Autodesk Fusion 360 part; units mm, degrees
note: some values were not read from the file. Chosen so that the rebuilt part matches the saved one: which bodies a step acts on.
(part 2 of 2)
sketch "Esquisse264" plane through (0, 25.75, 0) normal (0, 1, 0) x (1, 0, 0)
  spline S0 degree 5 poles (123.1631, -52) (123.1652, -52.1666) (123.167, -52.4997) (123.1624, -52.9994) (123.1419, -53.6656) (123.0924, -54.4971) (123.0197, -55.3268) (122.9244, -56.1541) (122.8078, -56.9784) (122.6713, -57.7994) (122.5162, -58.6168) (122.3444, -59.4305) (122.1576, -60.2403) (121.9575, -61.0465) (121.7457, -61.8491) (121.5239, -62.6484) (121.2935, -63.4447) (121.0557, -64.2383) (120.8113, -65.0295) (120.561, -65.8186) (120.305, -66.6056) (120.0432, -67.3906) (119.7752, -68.1736) (119.5004, -68.9543) (119.2175, -69.7325) (118.9255, -70.5075) (118.6227, -71.2788) (118.3076, -72.0454) (117.9784, -72.8065) (117.6337, -73.5608) (117.2717, -74.3073) (116.891, -75.0446) (116.4903, -75.7713) (116.0688, -76.4862) (115.6257, -77.188) (115.1609, -77.8756) (114.6743, -78.548) (114.1664, -79.2042) (113.638, -79.8439) (113.0901, -80.4668) (112.5241, -81.073) (111.9416, -81.6629) (111.3444, -82.2371) (110.7343, -82.7967) (110.1134, -83.3429) (109.4834, -83.8772) (108.8464, -84.4013) (108.2041, -84.9169) (107.558, -85.4257) (106.9097, -85.9295) (106.2604, -86.4299) (105.6109, -86.9284) (104.9621, -87.4261) (104.3142, -87.9239) (103.6674, -88.4223) (103.0212, -88.9214) (102.3753, -89.4209) (101.7287, -89.9203) (101.0804, -90.4184) (100.4293, -90.914) (99.7739, -91.4054) (99.113, -91.8906) (98.4451, -92.3676) (97.7689, -92.834) (97.0833, -93.2877) (96.3873, -93.7262) (95.6801, -94.1472) (94.9613, -94.5486) (94.2307, -94.9285) (93.4883, -95.2851) (92.7345, -95.617) (91.9699, -95.9233) (91.1952, -96.2031) (90.4115, -96.4564) (89.6197, -96.6831) (88.821, -96.8839) (88.0167, -97.0597) (87.2077, -97.2118) (86.3953, -97.3415) (85.5803, -97.4507) (84.7636, -97.541) (83.946, -97.6145) (83.128, -97.6729) (82.31, -97.7181) (81.4926, -97.7516) (80.6758, -97.7751) (79.8598, -97.7897) (79.0447, -97.7964) (78.2305, -97.7959) (77.4172, -97.7887) (76.6046, -97.7748) (75.7929, -97.7541) (74.9819, -97.7263) (74.1716, -97.6907) (73.3619, -97.6467) (72.5531, -97.5936) (71.7452, -97.5305) (70.9382, -97.4567) (70.1325, -97.3715) (69.3281, -97.2746) (68.5253, -97.1656) (67.7242, -97.0445) (66.925, -96.9115) (66.1277, -96.7671) (65.3324, -96.6119) (64.539, -96.4469) (63.7472, -96.2733) (62.9567, -96.0923) (62.1673, -95.9052) (61.3784, -95.7135) (60.5895, -95.5184) (59.8001, -95.3212) (59.0096, -95.1228) (58.2176, -94.9242) (57.4236, -94.7256) (56.6273, -94.5271) (55.8285, -94.3286) (55.0272, -94.1293) (54.2235, -93.9283) (53.4175, -93.7241) (52.6099, -93.515) (51.8012, -93.299) (50.9923, -93.074) (50.1843, -92.8374) (49.3785, -92.5869) (48.5762, -92.3199) (47.7791, -92.0339) (46.9891, -91.7265) (46.2081, -91.3954) (45.4384, -91.0386) (44.682, -90.6544) (43.9413, -90.2412) (43.2186, -89.798) (42.5161, -89.3242) (41.8356, -88.8198) (41.1791, -88.2852) (40.5481, -87.721) (39.9437, -87.1286) (39.3667, -86.5094) (38.8174, -85.8654) (38.2957, -85.1987) (37.801, -84.5115) (37.3323, -83.8062) (36.8885, -83.0852) (36.4679, -82.3507) (36.0687, -81.6049) (35.6891, -80.8497) (35.327, -80.0871) (34.9804, -79.3187) (34.6472, -78.5459) (34.3256, -77.7699) (34.014, -76.9918) (33.7107, -76.2123) (33.4147, -75.432) (33.1249, -74.6512) (32.8408, -73.8702) (32.5621, -73.0889) (32.2889, -72.3072) (32.0216, -71.5248) (31.7606, -70.7415) (31.5071, -69.9568) (31.2619, -69.1703) (31.0263, -68.3816) (30.8016, -67.5904) (30.5889, -66.7964) (30.3894, -65.9996) (30.2043, -65.1997) (30.0342, -64.397) (29.88, -63.5915) (29.742, -62.7836) (29.6203, -61.9735) (29.5147, -61.1616) (29.4248, -60.3484) (29.3498, -59.5343) (29.2889, -58.7196) (29.2409, -57.9048) (29.2045, -57.09) (29.1785, -56.2755) (29.1614, -55.4615) (29.152, -54.648) (29.1492, -53.835) (29.1519, -53.0225) (29.1594, -52.2104) (29.1712, -51.3986) (29.1871, -50.5868) (29.2075, -49.7751) (29.2327, -48.9632) (29.2636, -48.1512) (29.3012, -47.3389) (29.3471, -46.5266) (29.4027, -45.7142) (29.4697, -44.9022) (29.55, -44.0908) (29.6454, -43.2805) (29.7574, -42.4719) (29.8878, -41.6658) (30.0378, -40.8628) (30.2087, -40.0637) (30.4012, -39.2694) (30.6157, -38.4807) (30.8522, -37.6982) (31.1106, -36.9227) (31.3902, -36.1546) (31.6899, -35.3942) (32.0086, -34.6417) (32.3445, -33.897) (32.696, -33.1597) (33.0612, -32.4295) (33.4381, -31.7057) (33.8249, -30.9874) (34.2197, -30.2739) (34.6208, -29.5641) (35.0266, -28.8573) (35.436, -28.1524) (35.8481, -27.449) (36.2622, -26.7463) (36.6782, -26.044) (37.0962, -25.342) (37.5169, -24.6404) (37.941, -23.9395) (38.3697, -23.24) (38.8046, -22.5428) (39.2473, -21.849) (39.6995, -21.16) (40.1631, -20.4772) (40.6399, -19.8023) (41.1315, -19.1373) (41.6396, -18.4839) (42.1655, -17.8442) (42.7101, -17.22) (43.2744, -16.6132) (43.8585, -16.0254) (44.4627, -15.4582) (45.0866, -14.9127) (45.7296, -14.3898) (46.3906, -13.8899) (47.0685, -13.4132) (47.7617, -12.9594) (48.4688, -12.5277) (49.1882, -12.1171) (49.918, -11.7261) (50.6567, -11.3531) (51.4026, -10.9961) (52.1544, -10.653) (52.9105, -10.3217) (53.67, -10) (54.4317, -9.6858) (55.1948, -9.3772) (55.9588, -9.0725) (56.7232, -8.7704) (57.4878, -8.4697) (58.2526, -8.1697) (59.0177, -7.8702) (59.7834, -7.5712) (60.5501, -7.2733) (61.3183, -6.9772) (62.0887, -6.6842) (62.8619, -6.3956) (63.6384, -6.1132) (64.4189, -5.8386) (65.2038, -5.5739) (65.9935, -5.3208) (66.7884, -5.0813) (67.5885, -4.8571) (68.3938, -4.6498) (69.2042, -4.4609) (70.0193, -4.2916) (70.8388, -4.1428) (71.6622, -4.0151) (72.4889, -3.9091) (73.3183, -3.8247) (74.1498, -3.762) (74.9828, -3.7205) (75.8167, -3.6997) (76.651, -3.6991) (77.4851, -3.7178) (78.3187, -3.7552) (79.1513, -3.8105) (79.9827, -3.883) (80.8124, -3.9724) (81.6402, -4.0781) (82.4658, -4.2002) (83.2888, -4.3386) (84.1088, -4.4935) (84.9254, -4.6655) (85.738, -4.8554) (86.5459, -5.0638) (87.3485, -5.2919) (88.1448, -5.5408) (88.934, -5.8114) (89.7148, -6.105) (90.4861, -6.4225) (91.2468, -6.7647) (91.9955, -7.1324) (92.7311, -7.5257) (93.4524, -7.9448) (94.1585, -8.3893) (94.8483, -8.8585) (95.5213, -9.3516) (96.1772, -9.8672) (96.8158, -10.4035) (97.4375, -10.9587) (98.0428, -11.5306) (98.6326, -12.1168) (99.2081, -12.7151) (99.771, -13.3227) (100.323, -13.9373) (100.8662, -14.5562) (101.4027, -15.177) (101.9349, -15.7973) (102.4651, -16.4148) (102.9958, -17.0277) (103.5291, -17.6341) (104.067, -18.2325) (104.6112, -18.8221) (105.1629, -19.4021) (105.7229, -19.9724) (106.2918, -20.5332) (106.8693, -21.0853) (107.4551, -21.6301) (108.0481, -22.1691) (108.647, -22.7043) (109.2501, -23.2379) (109.8556, -23.7724) (110.4613, -24.3099) (111.065, -24.8528) (111.6646, -25.4033) (112.2577, -25.9634) (112.8421, -26.5348) (113.4156, -27.1189) (113.9762, -27.7168) (114.522, -28.3292) (115.0515, -28.9568) (115.5632, -29.5995) (116.0561, -30.2572) (116.5296, -30.9294) (116.9832, -31.6156) (117.417, -32.3148) (117.831, -33.0261) (118.2258, -33.7486) (118.6023, -34.4813) (118.9611, -35.223) (119.3035, -35.9729) (119.6304, -36.7301) (119.9428, -37.4938) (120.2416, -38.2634) (120.5276, -39.0383) (120.8014, -39.8182) (121.0634, -40.6028) (121.3137, -41.3918) (121.552, -42.1851) (121.7781, -42.9827) (121.9912, -43.7844) (122.1905, -44.5903) (122.375, -45.4003) (122.5434, -46.2142) (122.6945, -47.032) (122.827, -47.8535) (122.9396, -48.6782) (123.031, -49.5058) (123.1003, -50.3356) (123.1373, -51.0009) (123.1544, -51.5004) (123.161, -51.8334) (123.1631, -52) knots 0 0 0 0 0 0 0.00277778 0.00555556 0.00833333 0.01111111 0.01388889 0.01666667 0.01944444 0.02222222 0.025 0.02777778 0.03055556 0.03333333 0.03611111 0.03888889 0.04166667 0.04444444 0.04722222 0.05 0.05277778 0.05555556 0.05833333 0.06111111 0.06388889 0.06666667 0.06944444 0.07222222 0.075 0.07777778 0.08055556 0.08333333 0.08611111 0.08888889 0.09166667 0.09444444 0.09722222 0.1 0.10277778 0.10555556 0.10833333 0.11111111 0.11388889 0.11666667 0.11944444 0.12222222 0.125 0.12777778 0.13055556 0.13333333 0.13611111 0.13888889 0.14166667 0.14444444 0.14722222 0.15 0.15277778 0.15555556 0.15833333 0.16111111 0.16388889 0.16666667 0.16944444 0.17222222 0.175 0.17777778 0.18055556 0.18333333 0.18611111 0.18888889 0.19166667 0.19444444 0.19722222 0.2 0.20277778 0.20555556 0.20833333 0.21111111 0.21388889 0.21666667 0.21944444 0.22222222 0.225 0.22777778 0.23055556 0.23333333 0.23611111 0.23888889 0.24166667 0.24444444 0.24722222 0.25 0.25277778 0.25555556 0.25833333 0.26111111 0.26388889 0.26666667 0.26944444 0.27222222 0.275 0.27777778 0.28055556 0.28333333 0.28611111 0.28888889 0.29166667 0.29444444 0.29722222 0.3 0.30277778 0.30555556 0.30833333 0.31111111 0.31388889 0.31666667 0.31944444 0.32222222 0.325 0.32777778 0.33055556 0.33333333 0.33611111 0.33888889 0.34166667 0.34444444 0.34722222 0.35 0.35277778 0.35555556 0.35833333 0.36111111 0.36388889 0.36666667 0.36944444 0.37222222 0.375 0.37777778 0.38055556 0.38333333 0.38611111 0.38888889 0.39166667 0.39444444 0.39722222 0.4 0.40277778 0.40555556 0.40833333 0.41111111 0.41388889 0.41666667 0.41944444 0.42222222 0.425 0.42777778 0.43055556 0.43333333 0.43611111 0.43888889 0.44166667 0.44444444 0.44722222 0.45 0.45277778 0.45555556 0.45833333 0.46111111 0.46388889 0.46666667 0.46944444 0.47222222 0.475 0.47777778 0.48055556 0.48333333 0.48611111 0.48888889 0.49166667 0.49444444 0.49722222 0.5 0.50277778 0.50555556 0.50833333 0.51111111 0.51388889 0.51666667 0.51944444 0.52222222 0.525 0.52777778 0.53055556 0.53333333 0.53611111 0.53888889 0.54166667 0.54444444 0.54722222 0.55 0.55277778 0.55555556 0.55833333 0.56111111 0.56388889 0.56666667 0.56944444 0.57222222 0.575 0.57777778 0.58055556 0.58333333 0.58611111 0.58888889 0.59166667 0.59444444 0.59722222 0.6 0.60277778 0.60555556 0.60833333 0.61111111 0.61388889 0.61666667 0.61944444 0.62222222 0.625 0.62777778 0.63055556 0.63333333 0.63611111 0.63888889 0.64166667 0.64444444 0.64722222 0.65 0.65277778 0.65555556 0.65833333 0.66111111 0.66388889 0.66666667 0.66944444 0.67222222 0.675 0.67777778 0.68055556 0.68333333 0.68611111 0.68888889 0.69166667 0.69444444 0.69722222 0.7 0.70277778 0.70555556 0.70833333 0.71111111 0.71388889 0.71666667 0.71944444 0.72222222 0.725 0.72777778 0.73055556 0.73333333 0.73611111 0.73888889 0.74166667 0.74444444 0.74722222 0.75 0.75277778 0.75555556 0.75833333 0.76111111 0.76388889 0.76666667 0.76944444 0.77222222 0.775 0.77777778 0.78055556 0.78333333 0.78611111 0.78888889 0.79166667 0.79444444 0.79722222 0.8 0.80277778 0.80555556 0.80833333 0.81111111 0.81388889 0.81666667 0.81944444 0.82222222 0.825 0.82777778 0.83055556 0.83333333 0.83611111 0.83888889 0.84166667 0.84444444 0.84722222 0.85 0.85277778 0.85555556 0.85833333 0.86111111 0.86388889 0.86666667 0.86944444 0.87222222 0.875 0.87777778 0.88055556 0.88333333 0.88611111 0.88888889 0.89166667 0.89444444 0.89722222 0.9 0.90277778 0.90555556 0.90833333 0.91111111 0.91388889 0.91666667 0.91944444 0.92222222 0.925 0.92777778 0.93055556 0.93333333 0.93611111 0.93888889 0.94166667 0.94444444 0.94722222 0.95 0.95277778 0.95555556 0.95833333 0.96111111 0.96388889 0.96666667 0.96944444 0.97222222 0.975 0.97777778 0.98055556 0.98333333 0.98611111 0.98888889 0.99166667 0.99444444 0.99722222 1 1 1 1 1 1
  point P0 (122.9141, -56.1919)
  point P1 (122.137, -60.3115)
  point P2 (121.0252, -64.3324)
  point P3 (119.7355, -68.2824)
  point P4 (118.2513, -72.1684)
  point P5 (116.4062, -75.9059)
  point P6 (114.0475, -79.3414)
  point P7 (111.1943, -82.3706)
  point P8 (108.0426, -85.0426)
  point P9 (104.8186, -87.5365)
  point P10 (101.6136, -90.0082)
  point P11 (98.3445, -92.4339)
  point P12 (94.8623, -94.5948)
  point P13 (91.098, -96.2288)
  point P14 (87.1171, -97.2217)
  point P15 (83.0536, -97.6742)
  point P16 (79.0065, -97.7947)
  point P17 (75, -97.725)
  point P18 (71.0226, -97.4621)
  point P19 (67.0768, -96.9347)
  point P20 (63.1725, -96.1407)
  point P21 (59.2799, -95.1906)
  point P22 (55.3208, -94.2022)
  point P23 (51.2461, -93.143)
  point P24 (47.1442, -91.7822)
  point P25 (43.2669, -89.8181)
  point P26 (39.9148, -87.0852)
  point P27 (37.2554, -83.6715)
  point P28 (35.2234, -79.8519)
  point P29 (33.5951, -75.9051)
  point P30 (32.1745, -71.9699)
  point P31 (30.9308, -68.0399)
  point P32 (29.9728, -64.065)
  point P33 (29.3984, -60.0408)
  point P34 (29.1741, -56.0092)
  point P35 (29.1631, -52)
  point P36 (29.2718, -47.9993)
  point P37 (29.565, -43.9886)
  point P38 (30.2282, -40.0034)
  point P39 (31.4044, -36.1325)
  point P40 (33.0584, -32.4423)
  point P41 (34.9998, -28.9059)
  point P42 (37.0472, -25.4252)
  point P43 (39.1861, -21.9486)
  point P44 (41.5745, -18.5745)
  point P45 (44.3966, -15.5283)
  point P46 (47.6974, -13.0079)
  point P47 (51.3445, -11.0275)
  point P48 (55.1362, -9.4018)
  point P49 (58.9481, -7.8977)
  point P50 (62.7881, -6.4246)
  point P51 (66.7307, -5.1023)
  point P52 (70.8139, -4.1524)
  point P53 (75, -3.725)
  point P54 (79.2152, -3.8198)
  point P55 (83.3997, -4.3628)
  point P56 (87.5015, -5.3437)
  point P57 (91.4298, -6.8595)
  point P58 (95.0469, -9.0093)
  point P59 (98.2461, -11.7366)
  point P60 (101.0604, -14.7819)
  point P61 (103.6889, -17.8099)
  point P62 (106.3828, -20.6172)
  point P63 (109.2635, -23.2495)
  point P64 (112.2237, -25.9357)
  point P65 (115.0015, -28.9051)
  point P66 (117.3674, -32.2438)
  point P67 (119.2619, -35.89)
  point P68 (120.7698, -39.736)
  point P69 (121.9704, -43.7179)
  point P70 (122.8164, -47.8166)
ref_plane "Plan de construction31" through (0, 35.75, 0) normal (0, 1, 0) x (0, 0, 1)
sketch "Esquisse265" plane through (0, 35.75, 0) normal (0, 1, 0) x (1, 0, 0)
  circle A0 centre (75, -52) radius 43
loft "Biseau organique" cut profiles "Esquisse264", "Esquisse265" section 1 section 2 bodies 1
sketch "Esquisse266" plane through (0, 0, 0) normal (0, 1, 0) x (1, 0, 0)
  circle A0 centre (75, -52) radius 37
extrude "Tunnel circulaire (usinage)" cut sketch "Esquisse266" along normal blind 20 from surface at 35.75 bodies 1
sketch "Esquisse267" plane through (0, 0, 0) normal (0, 1, 0) x (1, 0, 0)
  circle A0 centre (75, -52) radius 45
  circle A1 centre (75, -52) radius 37
extrude "Gorge bandeau LED (usinage)" cut sketch "Esquisse267" along normal blind 14 from surface at 35.75 bodies 1
sketch "Esquisse268" plane through (0, 0, 0) normal (0, 1, 0) x (1, 0, 0)
  line L0 (3, 67) -> (147, 67)
  line L1 (147, 67) -> (147, 12)
  line L2 (147, 12) -> (3, 12)
  line L3 (3, 12) -> (3, 67)
extrude "Cavite - partie basse (usinage)" cut sketch "Esquisse268" along normal blind 81 from surface at 4 bodies 1
sketch "Esquisse269" plane through (0, 0, 0) normal (0, 0, 1) x (1, 0, 0)
  line L0 (3, 4) -> (147, 4)
  line L1 (147, 4) -> (147, 85)
  line L2 (147, 85) -> (3, 85)
  line L3 (3, 85) -> (3, 4)
  line L4 (57, 4) -> (93, 4)
  line L5 (93, 4) -> (93, 55.5)
  line L6 (93, 55.5) -> (57, 55.5)
  line L7 (57, 55.5) -> (57, 4)
extrude "Cavite - sous plafond (usinage)" cut sketch "Esquisse269" along normal blind 8 from surface at -12 contours L0 L1 L2 L3 L5 L6 L7 bodies 1
split "Separation portail / socle" by plane through (0, 0, 0) normal (0, 0, 1) bodies 1 makes body 2 at (67.1392, 40.7775, 104.0341)
sketch "Esquisse270" plane through (0, 0, 0) normal (0, 0, 1) x (1, 0, 0)
  line L0 (60, 32.5) -> (90, 32.5)
  line L1 (90, 32.5) -> (90, 52.5)
  line L2 (90, 52.5) -> (60, 52.5)
  line L3 (60, 52.5) -> (60, 32.5)
extrude "Tenon du portail (usinage)" add sketch "Esquisse270" along normal blind 6 from surface at -6 bodies 2
sketch "Esquisse271" plane through (0, 0, 0) normal (0, 0, 1) x (1, 0, 0)
  line L0 (59.6, 32.1) -> (90.4, 32.1)
  line L1 (90.4, 32.1) -> (90.4, 52.9)
  line L2 (90.4, 52.9) -> (59.6, 52.9)
  line L3 (59.6, 52.9) -> (59.6, 32.1)
extrude "Mortaise du socle (usinage)" cut sketch "Esquisse271" along normal blind 6 from surface at -6 bodies 1
sketch "Esquisse272" plane through (0, 0, 0) normal (0, 0, 1) x (1, 0, 0)
  circle A0 centre (65, 42.5) radius 1.7
  circle A1 centre (85, 42.5) radius 1.7
extrude "Vis - passage (usinage)" cut sketch "Esquisse272" along normal blind 6 from surface at -12 bodies 1
sketch "Esquisse273" plane through (0, 0, 0) normal (0, 0, 1) x (1, 0, 0)
  circle A0 centre (65, 42.5) radius 3.3
  circle A1 centre (85, 42.5) radius 3.3
extrude "Vis - lamage (usinage)" cut sketch "Esquisse273" along normal blind 3 from surface at -12 bodies 1
sketch "Esquisse274" plane through (0, 0, 0) normal (0, 0, 1) x (1, 0, 0)
  circle A0 centre (65, 42.5) radius 1.3
  circle A1 centre (85, 42.5) radius 1.3
extrude "Vis - taraudage portail (usinage)" cut sketch "Esquisse274" along normal blind 14 from surface at -6 bodies 2
sketch "Esquisse275" plane through (0, 0, 0) normal (0, 0, 1) x (1, 0, 0)
  circle A0 centre (75, 42.5) radius 4
extrude "Conduit cables LED (usinage)" cut sketch "Esquisse275" along normal blind 22 from surface at -13 bodies 2 1
sketch "Esquisse276" plane through (0, 0, 0) normal (0, 1, 0) x (1, 0, 0)
  circle A0 centre (75, -52) radius 42.75
  circle A1 centre (75, -52) radius 37.25
extrude "Cache diffusant LED (usinage)" add sketch "Esquisse276" along normal blind 1.2 from surface at 36 separate body makes body 3
sketch "Esquisse277" plane through (0, 0, 0) normal (0, 1, 0) x (1, 0, 0)
  circle A0 centre (75, -52) radius 41.25
  circle A1 centre (75, -52) radius 37.25
extrude "Cache diffusant - jupe (usinage)" add sketch "Esquisse277" along normal blind 12.3 from surface at 37.2 bodies 3
sketch "Esquisse278" plane through (0, 0, 0) normal (0, 1, 0) x (1, 0, 0)
  circle A0 centre (85, 56) radius 5
  circle A1 centre (125, 56) radius 2.5
  line L0 (17.5, 67) -> (30.5, 67)
  line L1 (30.5, 67) -> (30.5, 59)
  line L2 (30.5, 59) -> (17.5, 59)
  line L3 (17.5, 59) -> (17.5, 67)
extrude "Percages capteurs (usinage)" cut sketch "Esquisse278" along normal blind 4 bodies 1
sketch "Esquisse279" plane through (0, 0, 0) normal (0, 1, 0) x (1, 0, 0)
  circle A0 centre (85, 56) radius 6.5
extrude "Logement buzzer (usinage)" cut sketch "Esquisse279" along normal blind 2 from surface at 2 bodies 1
sketch "Esquisse280" plane through (0, 0, 0) normal (0, 1, 0) x (1, 0, 0)
  line L0 (78, 67) -> (92, 67)
  line L1 (92, 67) -> (92, 64)
  line L2 (92, 64) -> (78, 64)
  line L3 (78, 64) -> (78, 67)
  line L4 (78, 48) -> (92, 48)
  line L5 (92, 48) -> (92, 45)
  line L6 (92, 45) -> (78, 45)
  line L7 (78, 45) -> (78, 48)
extrude "Support buzzer - rails horizontaux (usinage)" add sketch "Esquisse280" along normal blind 12 from surface at 4 bodies 1
sketch "Esquisse281" plane through (0, 0, 0) normal (0, 0, 1) x (1, 0, 0)
  line L0 (14.8, 4) -> (17.8, 4)
  line L1 (17.8, 4) -> (17.8, 45.2)
  line L2 (17.8, 45.2) -> (14.8, 45.2)
  line L3 (14.8, 45.2) -> (14.8, 4)
  line L4 (30.2, 4) -> (33.2, 4)
  line L5 (33.2, 4) -> (33.2, 45.2)
  line L6 (33.2, 45.2) -> (30.2, 45.2)
  line L7 (30.2, 45.2) -> (30.2, 4)
  line L8 (14.8, 45.2) -> (33.2, 45.2)
  line L9 (33.2, 45.2) -> (33.2, 48.2)
  line L10 (33.2, 48.2) -> (14.8, 48.2)
  line L11 (14.8, 48.2) -> (14.8, 45.2)
extrude "Berceau IR - nervures au sol (usinage)" add sketch "Esquisse281" along normal blind 4 from surface at -67 bodies 1
sketch "Esquisse282" plane through (0, 0, 0) normal (0, 1, 0) x (1, 0, 0)
  line L0 (3.3, 66.7) -> (146.7, 66.7)
  line L1 (146.7, 66.7) -> (146.7, 4.3)
  line L2 (146.7, 4.3) -> (3.3, 4.3)
  line L3 (3.3, 4.3) -> (3.3, 66.7)
extrude "Couvercle arriere (usinage)" add sketch "Esquisse282" along normal blind 3 from surface at 82 separate body makes body 4
sketch "Esquisse283" plane through (0, 0, 0) normal (1, 0, 0) x (0, 0, -1)
  circle A0 centre (12, 83.5) radius 1.5
  circle A1 centre (35.5, 83.5) radius 1.5
  circle A2 centre (59, 83.5) radius 1.5
extrude "Ergots gauche" add sketch "Esquisse283" along normal blind 1.1 from surface at 2.5 bodies 4
extrude "Ergots droit" add sketch "Esquisse283" along normal blind 1.1 from surface at 146.7 bodies 4
sketch "Esquisse284" plane through (0, 0, 0) normal (1, 0, 0) x (0, 0, -1)
  circle A0 centre (12, 83.5) radius 1.9
  circle A1 centre (35.5, 83.5) radius 1.9
  circle A2 centre (59, 83.5) radius 1.9
extrude "Logements gauche" cut sketch "Esquisse284" along normal blind 1.2 from surface at 1.8 bodies 1
extrude "Logements droit" cut sketch "Esquisse284" along normal blind 1.2 from surface at 147 bodies 1
fillet "Conges angles du socle" radius 4 4 edges at (150, 85, -35) (0, 85, -35) (0, 0, -35) (150, 0, -35) on bodies 1
ref_plane "Plan de construction32" through (0, 0, -40) normal (0, 0, 1) x (1, 0, 0)
split "Coupe du socle en deux" by plane through (0, 0, -40) normal (0, 0, 1) bodies 1 makes body 5 at (130.1333, 45.9667, 0)
sketch "Esquisse287" plane through (0, 0, 0) normal (0, 0, 1) x (1, 0, 0)
  line L0 (0.8, 1.3) -> (149.2, 1.3)
  line L1 (149.2, 1.3) -> (149.2, 85)
  line L2 (149.2, 85) -> (0.8, 85)
  line L3 (0.8, 85) -> (0.8, 1.3)
  line L4 (2.2, 2.7) -> (147.8, 2.7)
  line L5 (147.8, 2.7) -> (147.8, 85)
  line L6 (147.8, 85) -> (2.2, 85)
  line L7 (2.2, 85) -> (2.2, 2.7)
extrude "Languette d emboitement (usinage)" add sketch "Esquisse287" along normal blind 4 from surface at -40 contours L0 L1 L2 L3 L4 L5 L7 bodies 1
sketch "Esquisse288" plane through (0, 0, 0) normal (0, 0, 1) x (1, 0, 0)
  line L0 (0.6, 1.1) -> (149.4, 1.1)
  line L1 (149.4, 1.1) -> (149.4, 85)
  line L2 (149.4, 85) -> (0.6, 85)
  line L3 (0.6, 85) -> (0.6, 1.1)
  line L4 (2.4, 2.9) -> (147.6, 2.9)
  line L5 (147.6, 2.9) -> (147.6, 85)
  line L6 (147.6, 85) -> (2.4, 85)
  line L7 (2.4, 85) -> (2.4, 2.9)
extrude "Rainure d emboitement (usinage)" cut sketch "Esquisse288" along normal blind 4.2 from surface at -40 contours L0 L1 L2 L3 L4 L5 L7 bodies 5
hidden bodies 2 3 4
named bodies: "Socle - partie basse", "Portail", "Cache diffusant LED", "Couvercle arriere", "Socle - partie haute"
